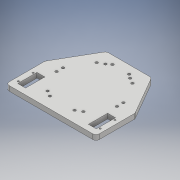
# Autodesk Inventor part: megapr
Saved by Autodesk Inventor 2018 (Build 220112000, 112)
## iProperties
Created: 2017-04-28
Part Number: megapr
Material: Generic
Document SubType Name: Modeling
Designer: cas13064
Density: 1 g/cm^3
Appearance: Default
Author: cas13064
Autodesk Inventor part; units mm, degrees
ref_plane "YZ Plane" through (0, 0, 0) normal (1, 0, 0) x (0, 1, 0)
ref_plane "XZ Plane" through (0, 0, 0) normal (0, 1, 0) x (-1, 0, 0)
ref_plane "XY Plane" through (0, 0, 0) normal (0, 0, 1) x (1, 0, 0)
sketch "Sketch1" plane through (0, 0, 0) normal (0, 0, 1) x (1, 0, 0)
  line L0 (0, 0) -> (0, 47.4625)
  line L1 (0, 47.4625) -> (27.4025, 94.925)
  line L2 (27.4025, 94.925) -> (82.2075, 94.925)
  line L3 (82.2075, 94.925) -> (109.61, 47.4625)
  line L4 (109.61, 47.4625) -> (109.61, 0)
  line L5 (109.61, 0) -> (0, 0)
  dimension "d2" = 54.805
  dimension "d3" = 120
  dimension "d4" = 120
  dimension "d5" = 47.4625
  dimension "d6" = 47.4625
  constraints: 12 end point, 2 equal length, 2 vertical, 1 horizontal, 1 perpendicular
  measures "d2" distance of L0.end L1.end
  measures "d3" angle of L2 L1
  measures "d4" angle of L3 L2
  measures "d5" vertical distance of L1.end L0.end
  measures "d6" distance of L0.start L0.end
extrude "Extrusion1" add sketch "Sketch1" along normal blind 6
sketch "Sketch2" plane through (0, 0, 6) normal (0, 0, 1) x (1, 0, 0)
  line L0 (0, 47.4625) -> (0, 0) projected
  line L1 (0, 0) -> (109.61, 0) projected
  line L2 (109.61, 0) -> (109.61, 47.4625) projected
  line L3 (109.61, 47.4625) -> (82.2075, 94.925) projected
  line L4 (82.2075, 94.925) -> (27.4025, 94.925) projected
  line L5 (27.4025, 94.925) -> (0, 47.4625) projected
  circle A0 centre (5, 28) radius 1.01
  circle A1 centre (5, 10) radius 1.01
  circle A2 centre (104.61, 28) radius 1.01
  circle A3 centre (104.61, 10) radius 1.01
  circle A4 centre (44.6125, 84.925) radius 1.6
  circle A5 centre (64.9975, 84.925) radius 1.6
  line L6 (7, 30.695) -> (16.57, 30.695)
  line L7 (16.57, 30.695) -> (16.57, 7.305)
  line L8 (16.57, 7.305) -> (7, 7.305)
  line L9 (7, 7.305) -> (7, 30.695)
  line L10 (93.04, 30.695) -> (102.61, 30.695)
  line L11 (102.61, 30.695) -> (102.61, 7.305)
  line L12 (102.61, 7.305) -> (93.04, 7.305)
  line L13 (93.04, 7.305) -> (93.04, 30.695)
  line L14 (82.2075, 94.925) -> (27.4025, 94.925) construction
  line L15 (54.805, 94.925) -> (54.805, 91.0637) construction
  line L16 (5, 28) -> (5, 10) construction
  line L17 (5, 19) -> (11.5154, 19) construction
  dimension "d10" = 2.02
  dimension "d11" = 3.2
  dimension "d12" = 5
  dimension "d13" = 5
  dimension "d14" = 18
  dimension "d15" = 10
  dimension "d16" = 23.39
  dimension "d17" = 9.57
  dimension "d19" = 2
  dimension "d20" = 2
  dimension "d21" = 20.385
  dimension "d22" = 10
  dimension "d23" = 3.8614
  constraints: 22 end point, 6 centre point, 4 equal radius, 4 horizontal alignment, 4 parallel, 3 horizontal, 2 equal length, 2 midpoint, 2 perpendicular, 2 vertical, 2 vertical alignment, 1 point on line, 1 symmetric about line, 1 other
  measures "d10" diameter of A0
  measures "d11" diameter of A4
  measures "d12" distance from line of L0 L16.start
  measures "d13" distance from line of L2 A2.centre
  measures "d14" distance of L16.end L16.start
  measures "d15" distance from line of L16.end L1
  measures "d16" distance of L6.end L7.end
  measures "d17" distance of L6.start L6.end
  measures "d19" distance from line of L16.end L9
  measures "d20" distance from line of A3.centre L11
  measures "d21" distance of A5.centre A4.centre
  measures "d22" distance from line of A4.centre L4
  measures "d23" distance of L15.start L15.end
extrude "Extrusion2" cut sketch "Sketch2" against normal through all contours A0 | A1 | A2 | A3 | A4 | A5 | L6 L7 L8 L9 | L10 L11 L12 L13
sketch "Sketch3" plane through (0, 0, 6) normal (0, 0, 1) x (1, 0, 0)
  line L0 (7, 7.305) -> (7, 30.695) projected
  line L1 (7, 30.695) -> (16.57, 30.695) projected
  line L2 (16.57, 30.695) -> (16.57, 7.305) projected
  line L3 (16.57, 7.305) -> (7, 7.305) projected
  circle A0 centre (44.6125, 84.925) radius 1.6 projected
  circle A1 centre (104.61, 28) radius 1.01 projected
  circle A2 centre (5, 28) radius 1.01 projected
  circle A3 centre (5, 10) radius 1.01 projected
  circle A4 centre (104.61, 10) radius 1.01 projected
  circle A5 centre (64.9975, 84.925) radius 1.6 projected
  line L4 (93.04, 7.305) -> (93.04, 30.695) projected
  line L5 (93.04, 30.695) -> (102.61, 30.695) projected
  line L6 (102.61, 30.695) -> (102.61, 7.305) projected
  line L7 (102.61, 7.305) -> (93.04, 7.305) projected
  line L8 (0, 47.4625) -> (0, 0) projected
  line L9 (0, 0) -> (109.61, 0) projected
  line L10 (109.61, 0) -> (109.61, 47.4625) projected
  line L11 (109.61, 47.4625) -> (82.2075, 94.925) projected
  line L12 (82.2075, 94.925) -> (27.4025, 94.925) projected
  line L13 (27.4025, 94.925) -> (0, 47.4625) projected
  line L14 (82.2075, 94.925) -> (109.61, 47.4625)
  line L15 (109.61, 47.4625) -> (82.2075, 0)
  line L16 (82.2075, 0) -> (27.4025, 0)
  line L17 (27.4025, 0) -> (0, 47.4625)
  line L18 (0, 47.4625) -> (27.4025, 94.925)
  line L19 (27.4025, 94.925) -> (82.2075, 94.925)
  circle A6 centre (33.055, 77.3404) radius 1.55
  circle A7 centre (39.805, 81.2375) radius 1.55
  circle A8 centre (69.805, 81.2375) radius 1.55
  circle A9 centre (18.055, 51.3596) radius 1.55
  circle A10 centre (18.055, 43.5654) radius 1.55
  circle A11 centre (33.055, 17.5846) radius 1.55
  circle A12 centre (39.805, 13.6875) radius 1.55
  circle A13 centre (69.805, 13.6875) radius 1.55
  circle A14 centre (76.555, 17.5846) radius 1.55
  circle A15 centre (91.555, 43.5654) radius 1.55
  circle A16 centre (91.555, 51.3596) radius 1.55
  line L20 (74.305, 81.2375) -> (93.805, 47.4625) construction
  line L21 (93.805, 47.4625) -> (74.305, 13.6875) construction
  line L22 (74.305, 13.6875) -> (35.305, 13.6875) construction
  line L23 (35.305, 13.6875) -> (15.805, 47.4625) construction
  line L24 (15.805, 47.4625) -> (35.305, 81.2375) construction
  line L25 (35.305, 81.2375) -> (74.305, 81.2375) construction
  circle A17 centre (76.555, 77.3404) radius 1.55
  point P0 (54.805, 47.4625)
  point P1 (54.805, 47.4625)
  dimension "d26" = 3.1
  dimension "d27" = 39
  dimension "d28" = 4.5
  dimension "d29" = 4.5
  dimension "d30" = 4.5
  dimension "d31" = 4.5
  dimension "d32" = 4.5
  dimension "d33" = 4.5
  dimension "d34" = 4.5
  dimension "d35" = 4.5
  dimension "d36" = 4.5
  dimension "d37" = 4.5
  dimension "d40" = 59.7557
  constraints: 24 end point, 12 centre point, 11 equal radius, 11 point on line, 2 vertical alignment, 1 coincident, 1 horizontal, 1 horizontal alignment, 26 other
  measures "d26" diameter of A6
  measures "d27" distance of L24.end L20.start
  measures "d28" distance of A7.centre L24.end
  measures "d29" distance of A6.centre L24.end
  measures "d30" distance of L20.start A8.centre
  measures "d31" distance of A9.centre L23.end
  measures "d32" distance of L23.end A10.centre
  measures "d33" distance of L22.end A11.centre
  measures "d34" distance of L20.end A16.centre
  measures "d35" distance of A15.centre L20.end
  measures "d36" distance of L21.end A14.centre
  measures "d37" distance of L20.start A17.centre
  measures "d40" distance of A11.centre A6.centre
extrude "Extrusion3" cut sketch "Sketch3" against normal through all contours A6 | A7 | A8 | A9 | A10 | A11 | A12 | A13 | A14 | A15 | A16 | A17
fillet "Fillet1" radius 4 6 edges at (109.61, 0, 3) (109.61, 47.4625, 3) (82.2075, 94.925, 3) (27.4025, 94.925, 3) (0, 47.4625, 3) (0, 0, 3)
equation "\"d4\" = d3"
equation "\"d6\" = d5"
equation "\"d13\" = d12"
equation "\"d20\" = d19"
equation "\"d29\" = d28"
equation "\"d30\" = d28"
equation "\"d31\" = d29"
equation "\"d32\" = d28"
equation "\"d33\" = d28"
equation "\"d34\" = d28"
equation "\"d35\" = d28"
equation "\"d36\" = d28"
equation "\"d37\" = d30"
body "Solid1"
